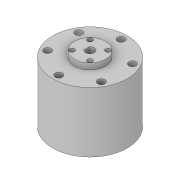
# Autodesk Inventor part: wheel insert
Saved by Autodesk Inventor 2020 (Build 240168000, 168)
## iProperties
Created: 2019-09-21
Part Number: wheel insert
Material: Generic
Document SubType Name: Modeling
Designer: ball
Density: 1 g/cm^3
Appearance: Default
Author: ball
Autodesk Inventor part; units mm, degrees
ref_plane "YZ Plane" through (0, 0, 0) normal (1, 0, 0) x (0, 1, 0)
ref_plane "XZ Plane" through (0, 0, 0) normal (0, 1, 0) x (-1, 0, 0)
ref_plane "XY Plane" through (0, 0, 0) normal (0, 0, 1) x (1, 0, 0)
sketch "Sketch1" plane through (0, 0, 0) normal (0, 1, 0) x (-1, 0, 0)
  circle A0 centre (145.0721, -68.2626) radius 28.4988
  arc A1 (147.6629, -66.2154) -> (147.6629, -70.3098) centre (145.0721, -68.2626) ccw
  line L0 (147.6629, -70.3098) -> (147.6629, -66.2154)
  circle A2 centre (144.9959, -92.0115) radius 2.794
  circle A3 centre (145.1103, -44.4477) radius 2.794
  circle A4 centre (165.6011, -80.2031) radius 2.794
  circle A5 centre (124.4669, -56.3221) radius 2.794
  circle A6 centre (165.6773, -56.4542) radius 2.794
  circle A7 centre (124.4287, -80.137) radius 2.794
  circle A8 centre (145.1483, -44.5137) radius 2.794
  circle A9 centre (145.0339, -92.0776) radius 2.794
  circle A10 centre (124.5431, -56.3222) radius 2.794
  circle A11 centre (165.6773, -80.2032) radius 2.794
  circle A12 centre (124.4669, -80.0711) radius 2.794
  circle A13 centre (165.7155, -56.3882) radius 2.794
  circle A14 centre (151.9123, -75.1789) radius 1.9685
  circle A15 centre (151.9884, -61.4224) radius 1.9685
  circle A16 centre (138.2319, -61.3463) radius 1.9685
  circle A17 centre (138.1558, -75.1028) radius 1.9685
  point P0 (0, 0)
  dimension "d1" = 6.604
  dimension "d3" = 5.588
  dimension "d4" = 23.749
  dimension "d7" = 360
  dimension "d9" = 3.937
  dimension "d14" = 360
  dimension "d25" = 2.5908
  constraints: 18 centre point, 2 end point, 2 point on circle, 1 coincident, 1 vertical, 34 other
  measures "d1" diameter of A1
  measures "d3" diameter of A2
  measures "d4" distance of A0.centre A2.centre
  measures "d9" diameter of A14
  measures "d25" distance from line of A0.centre L0
extrude "Extrusion1" add sketch "Sketch1" along normal blind 50.038 contours A0 | A2 A9 | A3 A8 | A4 A11 | A5 A10 | A6 A13 | A7 A12 picked at (146.4388, -94.4143) picked at (146.5538, -46.8501) picked at (168.4221, -80.4123) picked at (127.2879, -56.5313) picked at (167.123, -54.0531) picked at (125.875, -77.7363)
sketch "Sketch2" plane through (-145.0721, 50.038, -68.2626) normal (0, 1, 0) x (1, 0, 0)
  circle A0 centre (0, 0) radius 11.8872
  circle A1 centre (0, 0) radius 28.4988
  point P0 (145.0721, -68.2626)
  dimension "d18" = 23.7744
  constraints: 2 centre point, 1 coincident
  measures "d18" diameter of A0
extrude "Extrusion2" cut sketch "Sketch2" against normal blind 2.032
sketch "Sketch3" plane through (-145.0721, 0, -68.2626) normal (0, -1, 0) x (1, 0, 0)
  arc A0 (-2.5908, -2.0472) -> (-2.5908, 2.0472) centre (0, 0) ccw projected
  circle A1 centre (0, 0) radius 11.8872
  circle A2 centre (0, 0) radius 28.4988
  point P0 (145.0721, 68.2626)
  constraints: 2 centre point, 2 coincident
extrude "Extrusion3" cut sketch "Sketch3" against normal blind 2.032
sketch "Sketch4" plane through (-145.0721, 50.038, -68.2626) normal (0, 1, 0) x (1, 0, 0)
  circle A0 centre (0, 0) radius 11.8872 construction
  circle A1 centre (6.9163, 6.8402) radius 1.9685 construction
  circle A2 centre (-6.8402, 6.9163) radius 1.9685 construction
  circle A3 centre (-6.9163, -6.8402) radius 1.9685 construction
  circle A4 centre (6.8402, -6.9163) radius 1.9685 construction
  arc A5 (-2.5908, -2.0472) -> (-2.5908, 2.0472) centre (0, 0) ccw construction
  line L0 (-2.5908, -2.0472) -> (-2.5908, 2.0472) construction
  arc A6 (-2.5908, -2.0472) -> (-2.5908, 2.0472) centre (0, 0) ccw projected
  arc A7 (-2.5908, -2.0472) -> (-2.5908, 2.0472) centre (0, 0) ccw
  circle A8 centre (0, 0) radius 11.8872
  circle A9 centre (-6.8402, 6.9163) radius 1.9685
  circle A10 centre (6.9163, 6.8402) radius 1.9685 projected
  circle A11 centre (6.9163, 6.8402) radius 1.9685
  circle A12 centre (-6.9163, -6.8402) radius 1.9685
  circle A13 centre (6.8402, -6.9163) radius 1.9685
  line L1 (-2.5908, 2.0472) -> (-2.5908, -2.0472)
  point P0 (145.0721, -68.2626)
  constraints: 6 centre point, 6 coincident, 2 end point, 2 point on circle, 1 concentric, 1 vertical
extrude "Extrusion4" add sketch "Sketch4" along normal blind 2.54
body "Solid1"
